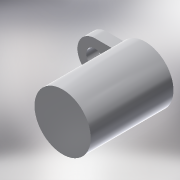
# Autodesk Inventor part: Tensioner
Saved by Autodesk Inventor 2018.2 (Build 222227000, 227)
## iProperties
Created: 2018-03-28
Part Number: Tensioner
Material: ABS Plastic
Document SubType Name: Modeling
Designer: Muchen He
Density: 1.06 g/cm^3
Appearance: Smooth - White
Author: Muchen He
Autodesk Inventor part; units mm, degrees
ref_plane "YZ Plane" through (0, 0, 0) normal (1, 0, 0) x (0, 1, 0)
ref_plane "XZ Plane" through (0, 0, 0) normal (0, 1, 0) x (-1, 0, 0)
ref_plane "XY Plane" through (0, 0, 0) normal (0, 0, 1) x (1, 0, 0)
sketch "Sketch1" plane through (0, 0, 0) normal (0, 1, 0) x (-1, 0, 0)
  circle A0 centre (0, 0) radius 1.5
  circle A1 centre (-6.5, 0) radius 4.7625
  line L0 (-2.8012, -3) -> (0, -3)
  arc A2 (0, -3) -> (0, 3) centre (0, 0) ccw
  line L1 (0, 3) -> (-2.8012, 3)
  dimension "d0" = 3
  dimension "d1" = 9.525
  dimension "d2" = 6.5
  dimension "d3" = 3
  constraints: 4 end point, 4 point on circle, 3 centre point, 2 tangent, 1 coincident, 1 concentric, 1 horizontal, 1 horizontal alignment, 1 parallel
  measures "d0" diameter of A0
  measures "d1" diameter of A1
  measures "d2" distance of A1.centre point (0, 0)
  measures "d3" radius of A2
extrude "Extrusion1" add sketch "Sketch1" along normal blind 2
extrude "Extrusion2" add sketch "Sketch1" against normal blind 12 contours A1
body "Solid1"
